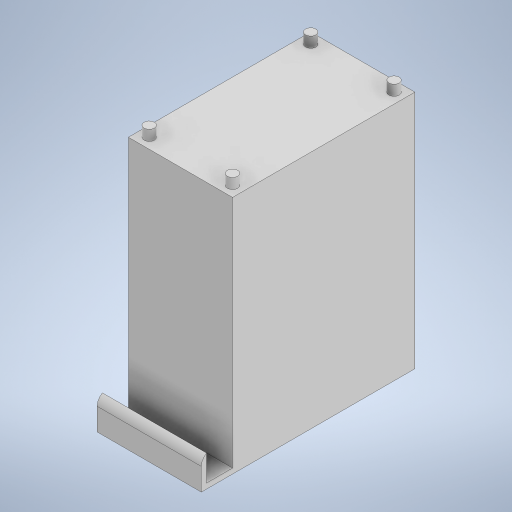
# Autodesk Inventor part: platform
Saved by Autodesk Inventor 2023.1 (Build 271208000, 208)
## iProperties
Created: 2023-05-29
Part Number: platform
Material: Generic
Document SubType Name: Modeling
Designer: Mansoor Lunawadi
Density: 1 g/cm^3
Appearance: Default
Author: Mansoor Lunawadi
Autodesk Inventor part; units mm, degrees
ref_plane "YZ Plane" through (0, 0, 0) normal (1, 0, 0) x (0, 1, 0)
ref_plane "XZ Plane" through (0, 0, 0) normal (0, 1, 0) x (-1, 0, 0)
ref_plane "XY Plane" through (0, 0, 0) normal (0, 0, 1) x (1, 0, 0)
sketch "Sketch1" plane through (0, 0, 0) normal (0, 1, 0) x (-1, 0, 0)
  line L0 (0, 0) -> (20, 0)
  line L1 (20, 0) -> (20, -35)
  line L2 (20, -35) -> (0, -35)
  line L3 (0, -35) -> (0, 0)
  dimension "d0" = 20
  dimension "d1" = 35
  constraints: 8 end point, 2 parallel, 1 horizontal, 1 perpendicular
  measures "d0" distance of L1.end L2.end
  measures "d1" distance of L0.end L1.end
extrude "Extrusion1" add sketch "Sketch1" along normal blind 46
sketch "Sketch2" plane through (-20, 0, 0) normal (0, 0, 1) x (1, 0, 0)
  line L0 (0, 0) -> (0, 46) projected
  line L1 (20, 0) -> (20, 46) projected
  line L2 (0, 0) -> (20, 0)
  line L3 (20, 0) -> (20, 1)
  line L4 (20, 1) -> (0, 1)
  line L5 (0, 1) -> (0, 0)
  dimension "d4" = 1
  constraints: 8 end point, 2 parallel, 1 horizontal, 1 perpendicular, 1 point on line
  measures "d4" distance of L3.end L2.end
extrude "Extrusion2" add sketch "Sketch2" along normal blind 6
sketch "Sketch3" plane through (-20, 1, 0) normal (0, 1, 0) x (1, 0, 0)
  line L0 (0, 35) -> (0, -6) projected
  line L1 (20, 35) -> (20, -6) projected
  line L2 (0, -6) -> (20, -6)
  line L3 (20, -6) -> (20, -5)
  line L4 (20, -5) -> (0, -5)
  line L5 (0, -5) -> (0, -6)
  point P0 (20, 0)
  dimension "d7" = 1
  constraints: 8 end point, 2 parallel, 1 horizontal, 1 perpendicular, 1 point on line
  measures "d7" distance of L3.end L2.end
extrude "Extrusion3" add sketch "Sketch3" along normal blind 5
fillet "Fillet1" radius 2 1 edges at (-10, 6, 6)
sketch "Sketch4" plane through (0, 46, 0) normal (0, 1, 0) x (1, 0, 0)
  arc A0 (-20, 2) -> (-18, 0) centre (-18, 2) ccw projected
  circle A1 centre (-18, 2) radius 1
  arc A2 (-2, 0) -> (0, 2) centre (-2, 2) ccw projected
  circle A3 centre (-2, 2) radius 1
  arc A4 (0, 33) -> (-2, 35) centre (-2, 33) ccw projected
  circle A5 centre (-2, 33) radius 1
  arc A6 (-18, 35) -> (-20, 33) centre (-18, 33) ccw projected
  circle A7 centre (-18, 33) radius 1
  point P0 (0, 0)
  dimension "d11" = 2
  dimension "d12" = 2
  dimension "d13" = 2
  dimension "d14" = 2
  constraints: 4 centre point, 4 coincident
  measures "d11" diameter of A1
  measures "d12" diameter of A3
  measures "d13" diameter of A5
  measures "d14" diameter of A7
extrude "Extrusion4" add sketch "Sketch4" along normal blind 2
body "Solid1"
